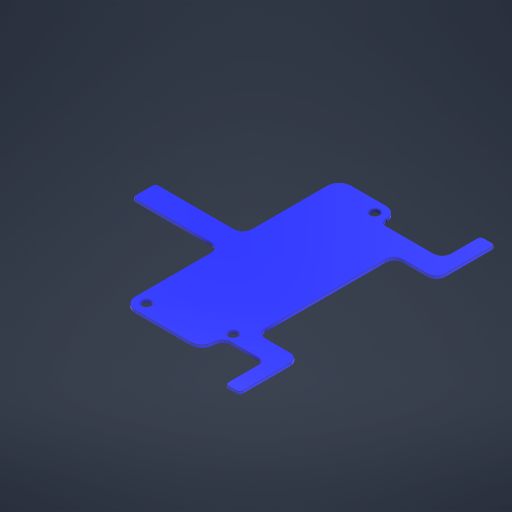
# Autodesk Inventor part: pcb
Saved by Autodesk Inventor 2024 (Build 280153000, 153)
## iProperties
Created: 2024-05-25
Part Number: pcb
Material: Generic
Document SubType Name: Modeling
Designer: Adam
Density: 1 g/cm^3
Appearance: Default
Author: Adam
Autodesk Inventor part; units mm, degrees
ref_plane "YZ Plane" through (0, 0, 0) normal (1, 0, 0) x (0, 1, 0)
ref_plane "XZ Plane" through (0, 0, 0) normal (0, 1, 0) x (-1, 0, 0)
ref_plane "XY Plane" through (0, 0, 0) normal (0, 0, 1) x (1, 0, 0)
ref_plane "Work Plane2" through (0, 1, 0) normal (0, 1, 0) x (1, 0, 0)
sketch "Sketch2" plane through (0, 1, 0) normal (0, 1, 0) x (1, 0, 0)
  line L0 (14.2983, 30.8418) -> (8.4694, 30.8418)
  line L1 (18.2983, -20.3933) -> (18.2983, 20.8418)
  line L2 (6.4694, 32.8418) -> (6.4694, 32.9551)
  line L3 (2.4694, 36.9551) -> (-9.8229, 36.9551)
  line L4 (-9.8229, -37.4026) -> (9.2983, -37.4026)
  line L5 (13.2983, -33.4026) -> (13.2983, -33.6636)
  arc A0 (9.2983, -37.4026) -> (13.2983, -33.4026) centre (9.2983, -33.4026) ccw
  arc A1 (-13.8229, -33.4026) -> (-9.8229, -37.4026) centre (-9.8229, -33.4026) ccw
  arc A2 (6.4694, 32.9551) -> (2.4694, 36.9551) centre (2.4694, 32.9551) ccw
  arc A3 (-9.8229, 36.9551) -> (-13.8229, 32.9551) centre (-9.8229, 32.9551) ccw
  arc A4 (6.4694, 32.8418) -> (8.4694, 30.8418) centre (8.4694, 32.8418) ccw
  circle A5 centre (2.4694, 32.9551) radius 1.55
  circle A6 centre (14.2983, -27.6636) radius 1.55
  circle A7 centre (-9.8229, -33.4026) radius 1.55
  line L6 (20.7089, 30.8418) -> (13.8839, 30.8418)
  line L7 (28.7927, 44.0538) -> (31.7927, 44.0538)
  line L8 (32.7927, 43.0538) -> (32.7927, 26.8418)
  line L9 (29.7927, 23.8418) -> (21.2983, 23.8418)
  line L10 (21.2983, -23.3933) -> (29.7927, -23.3933)
  line L11 (-16.8229, 3.7762) -> (-42.9549, 3.7762)
  line L12 (-43.9549, 2.7762) -> (-43.9549, -3.2238)
  line L13 (-42.9549, -4.2238) -> (-16.8229, -4.2238)
  arc A8 (15.8618, -30.3933) -> (13.2983, -33.4026) centre (16.3463, -33.4026) ccw
  line L14 (15.8618, -30.3933) -> (25.7927, -30.3933)
  line L15 (32.7927, -26.3933) -> (32.7927, -42.9467)
  line L16 (27.7927, -32.3933) -> (27.7927, -42.9467)
  line L17 (28.7927, -43.9467) -> (31.7927, -43.9467)
  line L18 (27.7927, 43.0538) -> (27.7927, 33.8418)
  line L19 (24.7927, 30.8418) -> (20.7089, 30.8418)
  line L20 (-13.8229, 32.9551) -> (-13.8229, 6.7762)
  line L21 (-13.8229, -7.2238) -> (-13.8229, -33.4026)
  arc A9 (28.7927, 44.0538) -> (27.7927, 43.0538) centre (28.7927, 43.0538) ccw
  arc A10 (32.7927, 43.0538) -> (31.7927, 44.0538) centre (31.7927, 43.0538) ccw
  arc A11 (31.7927, -43.9467) -> (32.7927, -42.9467) centre (31.7927, -42.9467) ccw
  arc A12 (27.7927, -42.9467) -> (28.7927, -43.9467) centre (28.7927, -42.9467) ccw
  arc A13 (29.7927, 23.8418) -> (32.7927, 26.8418) centre (29.7927, 26.8418) ccw
  arc A14 (24.7927, 30.8418) -> (27.7927, 33.8418) centre (24.7927, 33.8418) ccw
  arc A15 (27.7927, -32.3933) -> (25.7927, -30.3933) centre (25.7927, -32.3933) ccw
  arc A16 (-16.8229, 3.7762) -> (-13.8229, 6.7762) centre (-16.8229, 6.7762) ccw
  arc A17 (-13.8229, -7.2238) -> (-16.8229, -4.2238) centre (-16.8229, -7.2238) ccw
  arc A18 (18.2983, -20.3933) -> (21.2983, -23.3933) centre (21.2983, -20.3933) ccw
  arc A19 (32.7927, -26.3933) -> (29.7927, -23.3933) centre (29.7927, -26.3933) ccw
  arc A20 (21.2983, 23.8418) -> (18.2983, 20.8418) centre (21.2983, 20.8418) ccw
  arc A21 (-42.9549, 3.7762) -> (-43.9549, 2.7762) centre (-42.9549, 2.7762) ccw
  arc A22 (-43.9549, -3.2238) -> (-42.9549, -4.2238) centre (-42.9549, -3.2238) ccw
  point P0 (0, 0)
  point P1 (18.2983, -31.6636)
  point P2 (13.2983, -31.6636)
  point P3 (18.2983, 23.8418)
  point P4 (27.7927, 44.0538)
  point P5 (32.7927, 44.0538)
  point P6 (32.7927, 23.8418)
  point P7 (32.7927, -23.3933)
  point P8 (32.7927, -43.9467)
  point P9 (27.7927, -30.3933)
  point P10 (-13.8229, -4.2238)
  point P11 (-13.8229, -0.2238)
  point P12 (25.5455, -23.3933)
  point P13 (18.2983, -23.3933)
  point P14 (30.2927, -43.9467)
  dimension "d12" = 2
  dimension "d13" = 3.1
  dimension "d15" = 3.1
  dimension "d18" = 4
  dimension "d19" = 7
  dimension "d23" = 5
  dimension "d24" = 5
  dimension "d25" = 14.4944
  dimension "d26" = 1
  dimension "d27" = 3
  dimension "d28" = 2
  dimension "d29" = 3
  dimension "d30" = 3
  dimension "d31" = 3
  dimension "d32" = 1
  dimension "d33" = 20.212
  dimension "d34" = 20.5534
  constraints: 44 end point, 41 tangent, 40 point on circle, 23 centre point, 21 point on line, 11 perpendicular, 7 equal radius, 4 horizontal, 3 vertical, 2 midpoint, 1 coincident, 1 parallel
  measures "d12" radius of A4
  measures "d13" diameter of A5
  measures "d15" diameter of A7
  measures "d18" distance of point (-13.823, -0.224) point (-13.823, -4.224)
  measures "d19" distance between parallel lines of L9 L6
  measures "d23" distance between parallel lines of L15 L16
  measures "d24" distance between parallel lines of L8 L18
  measures "d25" distance of point (32.793, 23.842) point (18.298, 23.842)
  measures "d26" radius of A9
  measures "d27" radius of A13
  measures "d28" radius of A15
  measures "d29" radius of A16
  measures "d30" radius of A18
  measures "d31" radius of A20
  measures "d32" radius of A21
  measures "d33" distance between parallel lines of L9 L7
  measures "d34" distance from line of point (30.293, -43.947) L10
extrude "Extrusion2" add sketch "Sketch2" along normal blind 1
body "Solid2"
